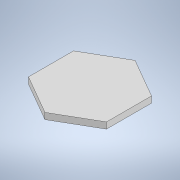
# Autodesk Inventor part: objeto5
Saved by Autodesk Inventor 2022.3 (Build 263350000, 350)
## iProperties
Created: 2023-06-18
Part Number: objeto5
Material: Generic
Document SubType Name: Modeling
Designer: crist
Density: 1 g/cm^3
Appearance: Default
Author: crist
Autodesk Inventor part; units mm, degrees
ref_plane "YZ Plane" through (0, 0, 0) normal (1, 0, 0) x (0, 1, 0)
ref_plane "XZ Plane" through (0, 0, 0) normal (0, 1, 0) x (-1, 0, 0)
ref_plane "XY Plane" through (0, 0, 0) normal (0, 0, 1) x (1, 0, 0)
sketch "Sketch1" plane through (0, 0, 0) normal (0, 1, 0) x (-1, 0, 0)
  circle A0 centre (0, 0) radius 25 construction
  line L0 (25, -14.4338) -> (0, -28.8675)
  line L1 (0, -28.8675) -> (-25, -14.4338)
  line L2 (-25, -14.4338) -> (-25, 14.4338)
  line L3 (-25, 14.4338) -> (0, 28.8675)
  line L4 (0, 28.8675) -> (25, 14.4338)
  line L5 (25, 14.4338) -> (25, -14.4338)
  point P0 (25, 0)
  dimension "d0" = 50
  constraints: 12 end point, 2 coincident, 1 horizontal alignment, 1 midpoint, 15 other
extrude "Extrusion1" add sketch "Sketch1" along normal blind 4
body "Solid1"
